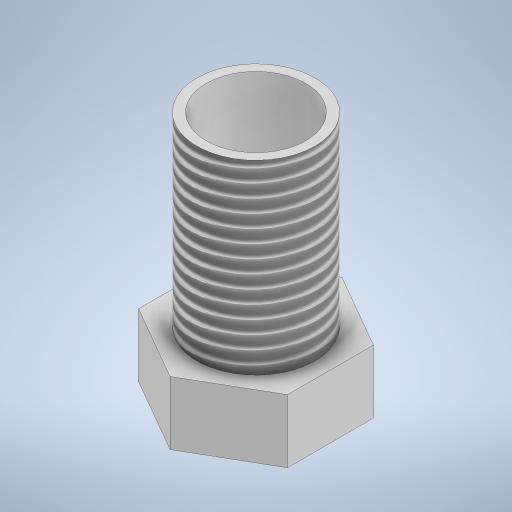
# Autodesk Inventor part: W9011M COAXIAL CONNECTOR
Saved by Autodesk Inventor 2023 (Build 270158000, 158)
## iProperties
Created: 2023-04-24
Part Number: W9011M COAXIAL CONNECTOR
Material: Generic
Document SubType Name: Modeling
Designer: Louis
Density: 1 g/cm^3
Appearance: Default
Author: Louis
Autodesk Inventor part; units mm, degrees
ref_plane "YZ Plane" through (0, 0, 0) normal (1, 0, 0) x (0, 1, 0)
ref_plane "XZ Plane" through (0, 0, 0) normal (0, 1, 0) x (-1, 0, 0)
ref_plane "XY Plane" through (0, 0, 0) normal (0, 0, 1) x (1, 0, 0)
sketch "Sketch1" plane through (0, 0, 0) normal (0, 0, 1) x (1, 0, 0)
  line L0 (0, 0) -> (3.175, 0)
  line L1 (3.175, 0) -> (3.175, 10)
  line L2 (3.175, 10) -> (0, 10)
  line L3 (0, 10) -> (0, 0)
  dimension "d0" = 3.175
  dimension "d1" = 10
  constraints: 8 end point, 2 parallel, 1 horizontal, 1 perpendicular
  measures "d0" distance of L1.end L2.end
  measures "d1" distance of L0.end L1.end
revolve "Revolution1" add sketch "Sketch1" angle 360 about axis through (0, 10, 0) along (0, -1, 0)
shell "Shell1" thickness 0.5 removed faces 1 at (0.8826, 10, -0.0433)
thread "Thread1" size "1/4-36 UNS" class "2A" standard "ANSI Unified Screw Threads" full length
sketch "Sketch2" plane through (0, 0, 0) normal (0, -1, 0) x (1, 0, 0)
  line L0 (0, 4.6188) -> (4, 2.3094)
  line L1 (4, 2.3094) -> (4, -2.3094)
  line L2 (4, -2.3094) -> (0, -4.6188)
  line L3 (0, -4.6188) -> (-4, -2.3094)
  line L4 (-4, -2.3094) -> (-4, 2.3094)
  line L5 (-4, 2.3094) -> (0, 4.6188)
  point P0 (0, 0)
  point P1 (0, 0)
  dimension "d6" = 8
  constraints: 12 end point, 1 coincident, 13 other
  measures "d6" distance between parallel lines of L1 L4
extrude "Extrusion1" add sketch "Sketch2" along normal blind 3.4
body "Solid1"
